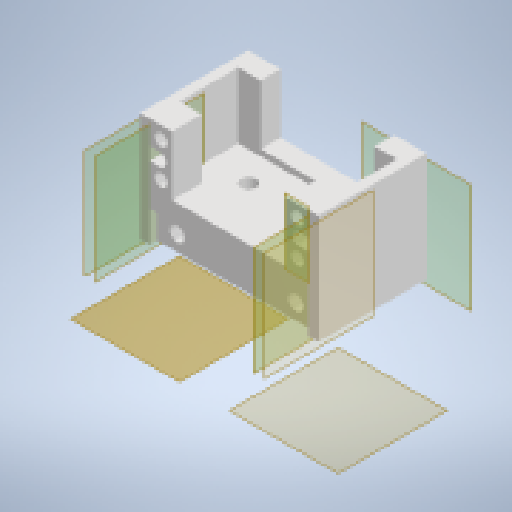
# Autodesk Inventor part: держатель сервомоторчика
Saved by Autodesk Inventor 2024.2 (Build 282272000, 272)
## iProperties
Created: 2025-11-28
Part Number: держатель сервомоторчика
Material: Типовые
Document SubType Name: Modeling
Designer: katya_notebook
Density: 1 g/cm^3
Appearance: По умолчанию
Author: katya_notebook
Autodesk Inventor part; units mm, degrees
ref_plane "YZ Plane" through (0, 0, 0) normal (1, 0, 0) x (0, 1, 0)
ref_plane "XZ Plane" through (0, 0, 0) normal (0, 1, 0) x (-1, 0, 0)
ref_plane "XY Plane" through (0, 0, 0) normal (0, 0, 1) x (1, 0, 0)
ref_plane "РабПлоскость1" through (0, 34.8975, 74.4992) normal (0, 0, -1) x (1, 0, 0)
sketch "Эскиз1" plane through (0, 34.8975, 74.4992) normal (0, 0, -1) x (1, 0, 0)
  line L0 (11.5, 6) -> (11.5, -6) projected
  line L1 (15, -6) -> (11.5, -6) projected
  arc A0 (15, -6) -> (16, -5) centre (15, -5) ccw projected
  line L2 (16, -1.25) -> (16, -5) projected
  line L3 (14, -1.25) -> (16, -1.25) projected
  arc A1 (12.8, -0.05) -> (14, -1.25) centre (14, -0.05) ccw projected
  line L4 (12.8, 0.05) -> (12.8, -0.05) projected
  arc A2 (14, 1.25) -> (12.8, 0.05) centre (14, 0.05) ccw projected
  line L5 (16, 1.25) -> (14, 1.25) projected
  line L6 (16, 5) -> (16, 1.25) projected
  arc A3 (16, 5) -> (15, 6) centre (15, 5) ccw projected
  line L7 (11.5, 6) -> (15, 6) projected
  circle A4 centre (13.75, 3.5) radius 1.25 projected
  circle A5 centre (13.75, -3.5) radius 1.25 projected
  line L8 (-11.5, -6) -> (-11.5, 6) projected
  line L9 (-15, 6) -> (-11.5, 6) projected
  arc A6 (-15, 6) -> (-16, 5) centre (-15, 5) ccw projected
  line L10 (-16, 1.3872) -> (-16, 5) projected
  line L11 (-14, 1.3872) -> (-16, 1.3872) projected
  arc A7 (-12.802, 0.1186) -> (-14, 1.3872) centre (-14, 0.1872) ccw projected
  line L12 (-12.802, 0.0186) -> (-12.802, 0.1186) projected
  arc A8 (-14, -1.25) -> (-12.802, 0.0186) centre (-14, -0.05) ccw projected
  line L13 (-16, -1.25) -> (-14, -1.25) projected
  line L14 (-16, -5) -> (-16, -1.25) projected
  arc A9 (-16, -5) -> (-15, -6) centre (-15, -5) ccw projected
  line L15 (-11.5, -6) -> (-15, -6) projected
  circle A10 centre (-13.75, 3.5) radius 1.25 projected
  circle A11 centre (-13.75, -3.5) radius 1.25 projected
  line L16 (16, 5) -> (16, 6)
  line L17 (16, 6) -> (15, 6)
  line L18 (-16, 5) -> (-16, 6)
  line L19 (-16, 6) -> (-15, 6)
  line L20 (16, -5) -> (16, -6)
  line L21 (16, -6) -> (15, -6)
  line L22 (-16, -5) -> (-16, -6)
  line L23 (-16, -6) -> (-15, -6)
  point P0 (0, 34.8975)
  constraints: 16 end point, 5 perpendicular, 3 point on line, 2 point on circle, 2 vertical
extrude "Выдавливание1" add sketch "Эскиз1" along normal blind 6
sketch "Эскиз3" plane through (11.5, 28.8975, 74.4992) normal (0, -1, 0) x (1, 0, 0)
  line L0 (-23, 0) -> (-23, -6) projected
  line L1 (-23, -6) -> (-23, 0)
  line L2 (-23, 0) -> (-27.5, 0)
  line L3 (0, -6) -> (-23, -6)
  line L4 (-23, -6) -> (-23, 0)
  line L5 (-23, 0) -> (0, 0)
  line L6 (-23, -6) -> (-27.5, -6) projected
  line L7 (-23, -6) -> (-27.5, -6)
  line L8 (-27.5, -6) -> (-27.5, 0)
  line L9 (0, 0) -> (4.5, 0)
  line L10 (0, -6) -> (0, 0)
  line L11 (4.5, 0) -> (4.5, -6)
  line L12 (4.5, -6) -> (0, -6)
  point P0 (-11.5, -74.4992)
  point P1 (4.5, 0)
  constraints: 22 end point, 3 horizontal, 3 perpendicular, 1 parallel, 1 vertical
extrude "Выдавливание2" add sketch "Эскиз3" along normal blind 30
ref_plane "РабПлоскость2" through (-11.5, 28.8975, 52.6492) normal (0, 0, -1) x (0, 1, 0)
ref_plane "РабПлоскость3" through (-11.5, 28.8975, 52.6492) normal (0, 0, -1) x (0, 1, 0)
ref_plane "РабПлоскость6" through (-16, 2.8975, 68.4992) normal (0, 1, 0) x (1, 0, 0)
ref_plane "РабПлоскость4" through (-15, 28.8975, 52.6492) normal (0, -1, 0) x (1, 0, 0)
ref_plane "РабПлоскость8" through (-16, 2.8975, 68.4992) normal (0, 1, 0) x (1, 0, 0)
ref_plane "РабПлоскость5" through (-16, 2.8975, 68.4992) normal (0, 1, 0) x (1, 0, 0)
ref_plane "РабПлоскость7" through (16, 28.8975, 74.4992) normal (1, 0, 0) x (0, 0, -1)
ref_plane "РабПлоскость9" through (16, 28.8975, 74.4992) normal (-1, 0, 0) x (0, 0, 1)
ref_plane "РабПлоскость10" through (-16, 28.8975, 74.4992) normal (-1, 0, 0) x (0, 0, 1)
sketch "Эскиз14" plane through (11.5, -1.1025, 74.4992) normal (0, -1, 0) x (1, 0, 0)
  circle A0 centre (-3.5, -11.925) radius 2 projected
  circle A1 centre (-19.5, -11.925) radius 2 projected
  circle A2 centre (-3.5, -11.925) radius 1.5
  circle A3 centre (-19.5, -11.925) radius 1.5
  point P0 (-11.5, -74.4992)
  dimension "d38" = 3
  dimension "d39" = 3
  constraints: 2 centre point, 2 coincident
  measures "d38" diameter of A2
  measures "d39" diameter of A3
extrude "Выдавливание12" add sketch "Эскиз14" against normal blind 4
ref_plane "РабПлоскость14" through (18, 28.8975, 74.4992) normal (1, 0, 0) x (0, 0, -1)
sketch "Эскиз15" plane through (18, 28.8975, 74.4992) normal (1, 0, 0) x (0, 0, -1)
  line L0 (1.45, -3.75) -> (1.45, -63.75) projected
  line L1 (-2.55, -3.75) -> (1.45, -3.75) projected
  line L2 (-2.55, -3.75) -> (1.45, -3.75)
  line L3 (1.45, -3.75) -> (1.45, -34.5952)
  line L4 (1.45, -34.5952) -> (-2.55, -34.5952)
  line L5 (-2.55, -34.5952) -> (-2.55, -3.75)
  point P0 (74.4992, -28.8975)
  constraints: 8 end point, 2 perpendicular, 1 horizontal, 1 point on line
extrude "Выдавливание13" cut sketch "Эскиз15" against normal blind 100
ref_plane "РабПлоскость13" through (16, 2.8975, 68.4992) normal (0, 1, 0) x (1, 0, 0)
ref_plane "РабПлоскость12" through (-18, 28.8975, 74.4992) normal (-1, 0, 0) x (0, 0, 1)
ref_plane "РабПлоскость11" through (16, 28.8975, 52.6492) normal (0, 0, -1) x (-1, 0, 0)
sketch "Эскиз18" plane through (16, 28.8975, 52.6492) normal (0, 0, -1) x (-1, 0, 0)
  circle A0 centre (4, -6.8) radius 1.5 projected
  circle A1 centre (28, -6.8) radius 1.5 projected
  point P0 (16, -28.8975)
extrude "Выдавливание16" cut sketch "Эскиз18" along normal mid plane 73
sketch "Эскиз19" plane through (0, 34.8975, 68.4992) normal (0, 0, -1) x (-1, 0, 0)
  line L0 (-16, -36) -> (16, -36) projected
  line L1 (16, -1.3872) -> (16, -36) projected
  line L2 (-16, -36) -> (16, -36)
  line L3 (16, -36) -> (16, -16)
  line L4 (16, -16) -> (-16, -16)
  line L5 (-16, -16) -> (-16, -36)
  point P0 (0, -34.8975)
  point P1 (11.5, -36)
  point P2 (16, -36)
  dimension "d57" = 20
  constraints: 8 end point, 2 parallel, 1 horizontal, 1 perpendicular, 1 point on line
  measures "d57" distance of L0.start L4.end
extrude "Выдавливание17" cut sketch "Эскиз19" along normal mid plane 200
sketch "Эскиз13" plane through (-16, 28.8975, 74.4992) normal (-1, 0, 0) x (0, 0, 1)
  line L0 (-21.85, 12) -> (0, 12)
  line L1 (0, 12) -> (0, -10)
  line L2 (0, -10) -> (-21.85, -10)
  line L3 (-21.85, -10) -> (-21.85, 12)
  line L4 (0, 4.6128) -> (0, -3.75) projected
  point P0 (-74.4992, -28.8975)
  point P1 (0, 12)
  point P2 (-21.85, -30)
  dimension "d60" = 21.85
  dimension "d61" = 22
  dimension "d62" = 0
  constraints: 8 end point, 2 parallel, 1 horizontal, 1 perpendicular
  measures "d60" distance of L0.start L0.end
  measures "d61" distance of L2.end L0.start
  measures "d62" distance between parallel lines of L1 L4
sketch "Эскиз10" plane through (16, 28.8975, 74.4992) normal (1, 0, 0) x (0, 0, -1)
  line L0 (0, 12) -> (21.85, 12)
  line L1 (21.85, 12) -> (21.85, -10)
  line L2 (21.85, -10) -> (0, -10)
  line L3 (0, -10) -> (0, 12)
  line L4 (0, 12) -> (6, 12) projected
  line L5 (0, 4.75) -> (0, -3.75) projected
  point P0 (74.4992, -28.8975)
  point P1 (21.85, -30)
  dimension "d63" = 21.85
  dimension "d64" = 22
  dimension "d65" = 0
  dimension "d66" = 0
  constraints: 8 end point, 2 parallel, 1 horizontal, 1 perpendicular
  measures "d63" distance of L0.start L0.end
  measures "d64" distance of L2.end L0.start
  measures "d65" distance between parallel lines of L4 L0
  measures "d66" distance between parallel lines of L5 L3
extrude "Выдавливание18" add sketch "Эскиз13" along normal blind 2
extrude "Выдавливание19" add sketch "Эскиз10" along normal blind 2
sketch "Эскиз20" plane through (-16, 18.8975, 52.6492) normal (0, -1, 0) x (1, 0, 0)
  line L0 (32, 4) -> (0, 4)
  line L1 (0, 4) -> (0, 15.85)
  line L2 (0, 15.85) -> (32, 15.85)
  line L3 (32, 15.85) -> (32, 4)
  line L4 (0, 0) -> (0, 15.85) projected
  line L5 (32, 15.85) -> (0, 15.85) projected
  circle A0 centre (24, 9.925) radius 1.5
  circle A1 centre (8, 9.925) radius 1.5
  point P0 (16, -52.6492)
  dimension "d71" = 32
  dimension "d72" = 11.85
  dimension "d73" = 0
  dimension "d74" = 0
  dimension "d75" = 3
  dimension "d76" = 3
  dimension "d77" = 8
  dimension "d78" = 8
  dimension "d79" = 5.925
  dimension "d80" = 5.925
  constraints: 8 end point, 2 centre point, 2 parallel, 1 horizontal, 1 perpendicular
  measures "d71" distance of L0.start L0.end
  measures "d72" distance of L0.end L1.end
  measures "d73" distance between parallel lines of L4 L1
  measures "d74" distance between parallel lines of L5 L2
  measures "d75" diameter of A0
  measures "d76" diameter of A1
  measures "d77" distance from line of L1 A1.centre
  measures "d78" distance from line of L3 A0.centre
  measures "d79" distance from line of L0 A0.centre
  measures "d80" distance from line of L0 A1.centre
extrude "Выдавливание20" add sketch "Эскиз20" against normal blind 8.75
sketch "Эскиз21" plane through (16, 28.8975, 74.4992) normal (-1, 0, 0) x (0, 0, 1)
  line L0 (-21.85, 12) -> (-17.85, 12)
  line L1 (-17.85, 12) -> (-17.85, -10)
  line L2 (-17.85, -10) -> (-21.85, -10)
  line L3 (-21.85, -10) -> (-21.85, 12)
  line L4 (-17.85, -10) -> (-21.85, -10) projected
  line L5 (-17.85, -10) -> (-17.85, -1.25) projected
  point P0 (-74.4992, -28.8975)
  point P1 (-19.85, -10)
  dimension "d83" = 4
  dimension "d84" = 22
  dimension "d85" = 0
  dimension "d86" = 0
  constraints: 8 end point, 2 parallel, 1 horizontal, 1 midpoint, 1 perpendicular
  measures "d83" distance of L1.end L2.end
  measures "d84" distance of L2.end L0.start
  measures "d85" distance from line of point (-19.85, -10) L4
  measures "d86" distance between parallel lines of L5 L1
extrude "Выдавливание21" add sketch "Эскиз21" along normal blind 32.5
sketch "Эскиз22" plane through (-18, 18.8975, 52.6492) normal (0, 0, -1) x (-1, 0, 0)
  line L0 (-29.5, 10) -> (-29.5, 22) projected
  line L1 (-6.5, 22) -> (-6.5, 10) projected
  line L2 (-29.5, 10) -> (-6.5, 10)
  line L3 (-6.5, 10) -> (-6.5, 22)
  line L4 (-6.5, 22) -> (-29.5, 22)
  line L5 (-29.5, 22) -> (-29.5, 10)
  point P0 (-18, -18.8975)
  constraints: 8 end point, 2 parallel, 1 horizontal, 1 perpendicular
extrude "Выдавливание22" cut sketch "Эскиз22" against normal blind 32.5
